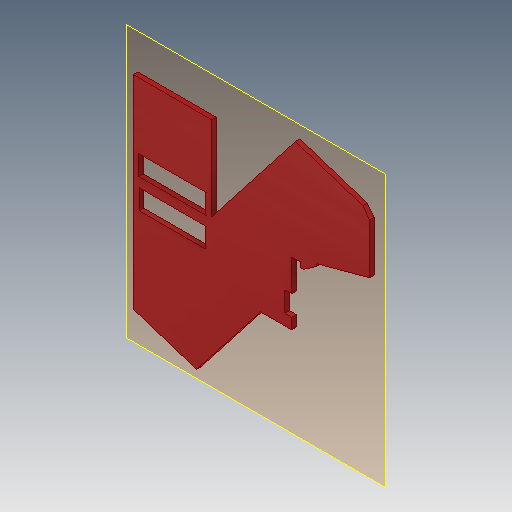
# Autodesk Inventor part: cellSTORM_v5_microscope_cover
Saved by Autodesk Inventor 2019.4 (Build 234330000, 330)
## iProperties
Created: 2020-04-27
Part Number: cellSTORM_v5_microscope_cover
Material: Generic
Document SubType Name: Modeling
Designer: diederichbenedict
Density: 1 g/cm^3
Appearance: Red
Author: diederichbenedict
Autodesk Inventor part; units mm, degrees
ref_plane "YZ Plane" through (0, 0, 0) normal (1, 0, 0) x (0, 1, 0)
ref_plane "XZ Plane" through (0, 0, 0) normal (0, 1, 0) x (-1, 0, 0)
ref_plane "XY Plane" through (0, 0, 0) normal (0, 0, 1) x (1, 0, 0)
ref_plane "Work Plane1" through (0, 0, 0) normal (0, 0, 1) x (1, 0, 0)
sketch "Sketch1" plane through (0, 0, 0) normal (0, 0, 1) x (1, 0, 0)
  line L0 (29.3421, 3.5361) -> (54.2162, 10.2011) projected
  line L1 (29.3421, 3.5361) -> (22.8734, 3.5361) projected
  line L2 (22.8734, 3.5361) -> (22.8734, -8.6704) projected
  line L3 (22.8734, -8.6704) -> (19.1468, -13.4402) projected
  line L4 (19.1468, -13.4402) -> (12.0348, -13.4402) projected
  line L5 (12.0348, -13.4402) -> (12.0348, -22.5432) projected
  line L6 (12.0348, -22.5432) -> (-14.689, -56.7481) projected
  line L7 (-14.689, -56.7481) -> (-41.2, -48.1342) projected
  line L8 (-41.2, -48.1342) -> (-41.2, -18.0876) projected
  line L9 (-41.2, -7.0876) -> (-38.2, -7.0876) projected
  line L10 (-38.2, -7.0876) -> (-38.2, -2.0876) projected
  line L11 (-38.2, -2.0876) -> (-41.4512, -2.0876) projected
  line L12 (-41.4512, -2.0876) -> (-41.4512, 5.4124) construction
  line L13 (-41.4512, 5.4124) -> (-41.2, 5.4124) construction
  line L14 (-41.2, 5.4124) -> (-41.2, 5.9124) construction
  line L15 (-41.2, 5.9124) -> (-38.2, 5.9124) projected
  line L16 (-38.2, 5.9124) -> (-38.2, 8.4124) projected
  line L17 (-38.2, 8.4124) -> (-41.2, 8.4124) projected
  line L18 (-41.2, 8.4124) -> (-41.2, 32.4124) projected
  line L19 (-41.2, 32.4124) -> (-12.4512, 32.4124) projected
  line L20 (-12.4512, 32.4124) -> (-12.4512, 8.4124) projected
  line L21 (-12.4512, 8.4124) -> (-15.4512, 8.4124) projected
  line L22 (-15.4512, 8.4124) -> (-15.4512, 5.9124) projected
  line L23 (-15.4512, 5.9124) -> (-12.4512, 5.9124) projected
  line L24 (-12.4512, 5.9124) -> (-12.4512, -2.0876) projected
  line L25 (-12.4512, -2.0876) -> (-15.4512, -2.0876) projected
  line L26 (-15.4512, -2.0876) -> (-15.4512, -7.0876) projected
  line L27 (-15.4512, -7.0876) -> (-12.4512, -7.0876) projected
  line L28 (-12.4512, -7.0876) -> (-12.4512, -15.0876) projected
  line L29 (-10.7358, -8.2808) -> (27.1735, 40.2407) projected
  line L30 (27.1735, 40.2407) -> (54.2162, 31.454) projected
  line L31 (54.2162, 31.454) -> (54.2162, 10.2011) projected
  line L32 (36.5437, 2.1484) -> (31.1264, -1.592) projected
  line L33 (36.5437, 2.1484) -> (37.0695, 3.5361) projected
  line L34 (60.3683, 9.779) -> (37.0695, 3.5361) projected
  line L35 (60.3683, 9.779) -> (60.3683, 9.784) projected
  line L36 (60.3683, 9.784) -> (60.3683, 25.084) projected
  line L37 (60.3683, 25.084) -> (60.3683, 31.9539) projected
  line L38 (60.3683, 31.9539) -> (57.3683, 35.9287) projected
  line L39 (57.3683, 35.9287) -> (27.5635, 45.6128) projected
  line L40 (27.5635, 45.6128) -> (-9.4512, -1.7639) projected
  line L41 (-9.4512, -1.7639) -> (-9.4512, 35.4124) projected
  line L42 (-9.4512, 35.4124) -> (-42.2, 35.4124) projected
  line L43 (-42.2, 35.4124) -> (-44.2, 35.4124) projected
  line L44 (-44.2, 35.4124) -> (-44.2, -54.5196) projected
  line L45 (-44.2, -54.5196) -> (-16.239, -63.6047) projected
  line L46 (-16.239, -63.6047) -> (12.0348, -27.416) projected
  line L47 (12.0348, -27.416) -> (25.8734, -27.416) projected
  line L48 (25.8734, -27.416) -> (25.8734, -22.5432) projected
  line L49 (25.8734, -22.5432) -> (22.8734, -22.5432) projected
  line L50 (22.8734, -22.5432) -> (22.8734, -13.5432) projected
  line L51 (22.8734, -13.5432) -> (25.8734, -13.5432) projected
  line L52 (25.8734, -13.5432) -> (25.8734, 0.5361) projected
  line L53 (25.8734, 0.5361) -> (29.5751, 0.5361) projected
  line L54 (29.5751, 0.5361) -> (29.5751, -1.592) projected
  line L55 (29.5751, -1.592) -> (31.1264, -1.592) projected
  line L56 (-12.4512, 5.9124) -> (-41.4512, 5.9124)
  line L57 (-41.4512, 5.9124) -> (-41.4512, -2.0876) construction
  line L58 (-41.4512, -2.0876) -> (-12.4512, -2.0876)
  line L59 (-12.4512, -2.0876) -> (-12.4512, 5.9124)
  line L60 (-12.4512, -7.0876) -> (-41.2, -7.0876)
  line L61 (-41.2, -7.0876) -> (-41.2, -15.0876)
  line L62 (-41.2, -15.0876) -> (-12.4512, -15.0876)
  line L63 (-12.4512, -15.0876) -> (-12.4512, -7.0876)
  line L64 (-41.4512, 5.9124) -> (-41.4512, -2.0876)
  line L65 (-41.2, -18.0876) -> (-38.2, -18.0876) projected
  line L66 (-38.2, -18.0876) -> (-38.2, -15.0876) projected
  line L67 (-38.2, -15.0876) -> (-41.2, -15.0876) projected
  line L68 (-41.2, -15.0876) -> (-41.2, -7.0876) projected
  line L69 (-12.4512, -15.0876) -> (-14.4512, -15.0876) projected
  line L70 (-14.4512, -15.0876) -> (-14.4512, -17.0876) projected
  line L71 (-14.4512, -17.0876) -> (-10.7358, -17.0876) projected
  line L72 (-10.7358, -17.0876) -> (-10.7358, -8.2808) projected
  point P0 (0, 0)
  dimension "d0" = 8
  constraints: 18 end point, 4 parallel, 2 horizontal, 2 perpendicular, 1 collinear, 1 point on line
  measures "d0" distance of L61.end L60.end
extrude "Extrusion1" add sketch "Sketch1" along normal blind 2 contours L1 L2 L3 L4 L5 L6 L7 L8 L65 L66 L62 L70 L71 L72 L29 L30 L31 L0 | L60 L10 L58 L26 | L56 L16 L17 L18 L19 L20 L21 L22 | L32 L55 L54 L53 L52 L51 L50 L49 L48 L47 L46 L45 L44 L43 L42 L41 L40 L39 L38 L37 L36 L35 L34 L33
sketch "Sketch2" plane through (0, 0, 0) normal (0, 0, -1) x (-1, 0, 0)
  line L0 (12.4512, -15.0876) -> (12.4512, -7.0876) projected
  line L1 (12.4512, -7.0876) -> (41.2, -7.0876) projected
  line L2 (41.2, -7.0876) -> (41.2, -15.0876) projected
  line L3 (41.2, -15.0876) -> (12.4512, -15.0876) projected
  line L4 (41.4512, 5.9124) -> (41.4512, -2.0876) projected
  line L5 (41.4512, -2.0876) -> (12.4512, -2.0876) projected
  line L6 (12.4512, -2.0876) -> (12.4512, 5.9124) projected
  line L7 (12.4512, 5.9124) -> (41.4512, 5.9124) projected
  line L8 (-36.5437, 2.1484) -> (-31.1264, -1.592) projected
  line L9 (-31.1264, -1.592) -> (-29.5751, -1.592) projected
  line L10 (-29.5751, -1.592) -> (-29.5751, 0.5361) projected
  line L11 (-29.5751, 0.5361) -> (-25.8734, 0.5361) projected
  line L12 (-25.8734, 0.5361) -> (-25.8734, -13.5432) projected
  line L13 (-25.8734, -13.5432) -> (-22.8734, -13.5432) projected
  line L14 (-22.8734, -13.5432) -> (-22.8734, -22.5432) projected
  line L15 (-22.8734, -22.5432) -> (-25.8734, -22.5432) projected
  line L16 (-25.8734, -22.5432) -> (-25.8734, -27.416) projected
  line L17 (-25.8734, -27.416) -> (-12.0348, -27.416) projected
  line L18 (-12.0348, -27.416) -> (16.239, -63.6047) projected
  line L19 (16.239, -63.6047) -> (44.2, -54.5196) projected
  line L20 (44.2, -54.5196) -> (44.2, 35.4124) projected
  line L21 (44.2, 35.4124) -> (9.4512, 35.4124) projected
  line L22 (9.4512, 35.4124) -> (9.4512, -1.7639) projected
  line L23 (9.4512, -1.7639) -> (-27.5635, 45.6128) projected
  line L24 (-27.5635, 45.6128) -> (-57.3683, 35.9287) projected
  line L25 (-57.3683, 35.9287) -> (-60.3683, 31.9539) projected
  line L26 (-60.3683, 31.9539) -> (-60.3683, 9.784) projected
  line L27 (-60.3683, 9.784) -> (-60.3683, 9.779) projected
  line L28 (-60.3683, 9.779) -> (-37.0695, 3.5361) projected
  line L29 (-37.0695, 3.5361) -> (-36.5437, 2.1484) projected
  line L30 (-29.3421, 3.5361) -> (-54.2162, 10.2011) projected
  line L31 (-54.2162, 10.2011) -> (-54.2162, 31.454) projected
  line L32 (-54.2162, 31.454) -> (-27.1735, 40.2407) projected
  line L33 (-27.1735, 40.2407) -> (10.7358, -8.2808) projected
  line L34 (12.4512, -15.0876) -> (12.4512, -7.0876) projected
  line L35 (12.4512, -7.0876) -> (15.4512, -7.0876) projected
  line L36 (15.4512, -7.0876) -> (15.4512, -2.0876) projected
  line L37 (15.4512, -2.0876) -> (12.4512, -2.0876) projected
  line L38 (12.4512, -2.0876) -> (12.4512, 5.9124) projected
  line L39 (12.4512, 5.9124) -> (15.4512, 5.9124) projected
  line L40 (15.4512, 5.9124) -> (15.4512, 8.4124) projected
  line L41 (15.4512, 8.4124) -> (12.4512, 8.4124) projected
  line L42 (12.4512, 8.4124) -> (12.4512, 32.4124) projected
  line L43 (12.4512, 32.4124) -> (41.2, 32.4124) projected
  line L44 (41.2, 32.4124) -> (41.2, 8.4124) projected
  line L45 (41.2, 8.4124) -> (38.2, 8.4124) projected
  line L46 (38.2, 8.4124) -> (38.2, 5.9124) projected
  line L47 (38.2, 5.9124) -> (41.2, 5.9124) projected
  line L48 (41.2, 5.9124) -> (41.2, 5.4124) projected
  line L49 (41.2, 5.4124) -> (41.4512, 5.4124) projected
  line L50 (41.4512, 5.4124) -> (41.4512, -2.0876) projected
  line L51 (41.4512, -2.0876) -> (38.2, -2.0876) projected
  line L52 (38.2, -2.0876) -> (38.2, -7.0876) projected
  line L53 (38.2, -7.0876) -> (41.2, -7.0876) projected
  line L54 (41.2, -18.0876) -> (41.2, -48.1342) projected
  line L55 (41.2, -48.1342) -> (14.689, -56.7481) projected
  line L56 (14.689, -56.7481) -> (-12.0348, -22.5432) projected
  line L57 (-12.0348, -22.5432) -> (-12.0348, -13.4402) projected
  line L58 (-12.0348, -13.4402) -> (-19.1468, -13.4402) projected
  line L59 (-19.1468, -13.4402) -> (-22.8734, -8.6704) projected
  line L60 (-22.8734, -8.6704) -> (-22.8734, 3.5361) projected
  line L61 (-22.8734, 3.5361) -> (-29.3421, 3.5361) projected
  circle A0 centre (37.2, 11.8299) radius 1.45 projected
  circle A1 centre (16.4512, 11.8299) radius 1.45 projected
  line L62 (12.6512, -7.0876) -> (12.6512, -11.0573)
  line L63 (12.6512, -11.0573) -> (-27.2448, 40.0073)
  line L64 (-27.2448, 40.0073) -> (-54.0162, 31.3087)
  line L65 (-54.0162, 31.3087) -> (-54.0162, 10.3546)
  line L66 (-54.0162, 10.3546) -> (-29.3158, 3.7361)
  line L67 (-29.3158, 3.7361) -> (-22.6734, 3.7361)
  line L68 (-22.6734, 3.7361) -> (-22.6734, -8.6016)
  line L69 (-22.6734, -8.6016) -> (-19.0493, -13.2402)
  line L70 (-19.0493, -13.2402) -> (-11.8348, -13.2402)
  line L71 (-11.8348, -13.2402) -> (-11.8348, -22.4744)
  line L72 (-11.8348, -22.4744) -> (14.7604, -56.5146)
  line L73 (14.7604, -56.5146) -> (41, -47.9889)
  line L74 (41, -47.9889) -> (41, -7.0876)
  line L75 (12.2936, -10.5996) -> (12.2936, -15.3176)
  line L76 (12.2936, -15.3176) -> (41, -15.3176)
  line L77 (12.6512, 32.3124) -> (41, 32.3124)
  line L78 (41, 32.3124) -> (41, 24.3283)
  line L79 (41, 24.3283) -> (12.6512, 24.3283)
  line L80 (12.6512, 24.3283) -> (12.6512, 32.3124)
  line L81 (41.2, -15.0876) -> (38.2, -15.0876) projected
  line L82 (38.2, -15.0876) -> (38.2, -18.0876) projected
  line L83 (38.2, -18.0876) -> (41.2, -18.0876) projected
  line L84 (10.7358, -8.2808) -> (10.7358, -17.0876) projected
  line L85 (10.7358, -17.0876) -> (14.4512, -17.0876) projected
  line L86 (14.4512, -17.0876) -> (14.4512, -15.0876) projected
  line L87 (14.4512, -15.0876) -> (12.4512, -15.0876) projected
  line L88 (41.2, -7.0876) -> (41.2, -15.0876) projected
  point P0 (0, 0)
  point P1 (12.4512, -10.4765)
  dimension "d3" = 0.2
  dimension "d4" = 7.9841
  dimension "d5" = 0.2
  dimension "d6" = 0.2
  dimension "d7" = 0.1
  constraints: 38 end point, 2 parallel, 2 perpendicular, 2 point on line, 1 horizontal, 1 vertical, 12 other
  measures "d3" distance between parallel lines of L31 L65
  measures "d4" distance of L79.end L77.start
  measures "d5" distance between parallel lines of L80 L42
  measures "d6" distance between parallel lines of L44 L78
  measures "d7" distance between parallel lines of L43 L77
extrude "Extrusion2" add sketch "Sketch2" along normal blind 2 contours L0 L63 L62 L1 L74 L3 | L0 L1 L62 L63 | L3 L82 L76 L86 | L76 L82 L83 L74 L73 L72 L71 L70 L69 L68 L67 L66 L65 L64 L63 L84 L85 L86 | L63 L64 L65 L66 L67 L68 L69 L70 L71 L72 L73 L74 L83 L54 L55 L56 L57 L58 L59 L60 L61 L30 L31 L32 L33 L84 | L74 L1 L2 L3 | L36 L5 L52 L1 | L77 L78 L79 L80
sketch "Sketch3" plane through (0, 0, -2) normal (0, 0, -1) x (-1, 0, 0)
  line L0 (12.4512, -7.0876) -> (12.4512, -15.0876) projected
  line L1 (10.7358, -8.2808) -> (-27.1735, 40.2407) projected
  line L2 (-27.1735, 40.2407) -> (-54.2162, 31.454) projected
  line L3 (-54.2162, 31.454) -> (-54.2162, 10.2011) projected
  line L4 (-54.2162, 10.2011) -> (-29.3421, 3.5361) projected
  line L5 (-29.3421, 3.5361) -> (-22.8734, 3.5361) projected
  line L6 (-22.8734, 3.5361) -> (-22.8734, -8.6704) projected
  line L7 (-22.8734, -8.6704) -> (-19.1468, -13.4402) projected
  line L8 (-19.1468, -13.4402) -> (-12.0348, -13.4402) projected
  line L9 (-12.0348, -13.4402) -> (-12.0348, -22.5432) projected
  line L10 (-12.0348, -22.5432) -> (14.689, -56.7481) projected
  line L11 (14.689, -56.7481) -> (41.2, -48.1342) projected
  line L12 (41.2, -15.0876) -> (41.2, -7.0876) projected
  line L13 (41.2, -7.0876) -> (38.2, -7.0876) projected
  line L14 (38.2, -7.0876) -> (38.2, -2.0876) projected
  line L15 (38.2, -2.0876) -> (15.4512, -2.0876) projected
  line L16 (15.4512, -2.0876) -> (15.4512, -7.0876) projected
  line L17 (15.4512, -7.0876) -> (12.4512, -7.0876) projected
  line L18 (38.2, -45.9545) -> (15.7598, -53.2458)
  line L19 (15.7598, -53.2458) -> (-9.0348, -21.5102)
  line L20 (-9.0348, -21.5102) -> (-9.0348, -10.4402)
  line L21 (-9.0348, -10.4402) -> (-17.6836, -10.4402)
  line L22 (-17.6836, -10.4402) -> (-19.8734, -7.6374)
  line L23 (-19.8734, -7.6374) -> (-19.8734, 6.5361)
  line L24 (-19.8734, 6.5361) -> (-28.9472, 6.5361)
  line L25 (-28.9472, 6.5361) -> (-51.2162, 12.5031)
  line L26 (-51.2162, 12.5031) -> (-51.2162, 29.2744)
  line L27 (-51.2162, 29.2744) -> (-28.2442, 36.7384)
  line L28 (-28.2442, 36.7384) -> (15.4512, -19.1891)
  line L29 (15.4512, -19.1891) -> (15.4512, -10.0876)
  line L30 (15.4512, -10.0876) -> (18.4512, -10.0876)
  line L31 (18.4512, -10.0876) -> (18.4512, -5.0876)
  line L32 (18.4512, -5.0876) -> (35.2, -5.0876)
  line L33 (35.2, -5.0876) -> (35.2, -10.0876)
  line L34 (35.2, -10.0876) -> (38.2, -10.0876)
  line L35 (38.2, -10.0876) -> (38.2, -45.9545)
  line L36 (12.4512, -15.0876) -> (14.4512, -15.0876) projected
  line L37 (14.4512, -15.0876) -> (14.4512, -17.0876) projected
  line L38 (14.4512, -17.0876) -> (10.7358, -17.0876) projected
  line L39 (10.7358, -17.0876) -> (10.7358, -8.2808) projected
  line L40 (41.2, -48.1342) -> (41.2, -18.0876) projected
  line L41 (41.2, -18.0876) -> (38.2, -18.0876) projected
  line L42 (38.2, -18.0876) -> (38.2, -15.0876) projected
  line L43 (38.2, -15.0876) -> (41.2, -15.0876) projected
  point P0 (0, 0)
  dimension "d10" = 3
  constraints: 36 end point, 17 other
  measures "d10" distance between parallel lines of L11 L18
extrude "Extrusion3" cut sketch "Sketch3" against normal up to surface (2 mm away) contours L38 L39 L28 | L28 L29 L30 L31 L32 L33 L34 L35 L18 L19 L20 L21 L22 L23 L24 L25 L26 L27 L39 L38
sketch "Sketch4" plane through (0, 0, 2) normal (0, 0, 1) x (1, 0, 0)
  line L0 (-12.4512, -7.0876) -> (-12.4512, -15.0876) projected
  line L1 (-12.4512, -15.0876) -> (-41.2, -15.0876) projected
  line L2 (-41.2, -15.0876) -> (-41.2, -7.0876) projected
  line L3 (-41.2, -7.0876) -> (-12.4512, -7.0876) projected
  line L4 (-41.4512, -2.0876) -> (-41.4512, 5.9124) projected
  line L5 (-41.4512, 5.9124) -> (-12.4512, 5.9124) projected
  line L6 (-12.4512, 5.9124) -> (-12.4512, -2.0876) projected
  line L7 (-12.4512, -2.0876) -> (-41.4512, -2.0876) projected
  line L8 (31.1264, -1.592) -> (36.5437, 2.1484) projected
  line L9 (36.5437, 2.1484) -> (37.0695, 3.5361) projected
  line L10 (37.0695, 3.5361) -> (60.3683, 9.779) projected
  line L11 (60.3683, 9.779) -> (60.3683, 9.784) projected
  line L12 (60.3683, 9.784) -> (60.3683, 31.9539) projected
  line L13 (60.3683, 31.9539) -> (57.3683, 35.9287) projected
  line L14 (57.3683, 35.9287) -> (27.5635, 45.6128) projected
  line L15 (27.5635, 45.6128) -> (-9.4512, -1.7639) projected
  line L16 (-9.4512, -1.7639) -> (-9.4512, 35.4124) projected
  line L17 (-9.4512, 35.4124) -> (-44.2, 35.4124) projected
  line L18 (-44.2, 35.4124) -> (-44.2, -54.5196) projected
  line L19 (-44.2, -54.5196) -> (-16.239, -63.6047) projected
  line L20 (-16.239, -63.6047) -> (12.0348, -27.416) projected
  line L21 (12.0348, -27.416) -> (25.8734, -27.416) projected
  line L22 (25.8734, -27.416) -> (25.8734, -22.5432) projected
  line L23 (25.8734, -22.5432) -> (22.8734, -22.5432) projected
  line L24 (22.8734, -22.5432) -> (22.8734, -13.5432) projected
  line L25 (22.8734, -13.5432) -> (25.8734, -13.5432) projected
  line L26 (25.8734, -13.5432) -> (25.8734, 0.5361) projected
  line L27 (25.8734, 0.5361) -> (29.5751, 0.5361) projected
  line L28 (29.5751, 0.5361) -> (29.5751, -1.592) projected
  line L29 (29.5751, -1.592) -> (31.1264, -1.592) projected
  line L30 (-41.6, -6.6876) -> (-41.6, -15.4876)
  line L31 (-41.6, -15.4876) -> (-12.0512, -15.4876)
  line L32 (-12.0512, -15.4876) -> (-12.0512, -6.6876)
  line L33 (-12.0512, -6.6876) -> (-41.6, -6.6876)
  line L34 (-41.8512, 6.3124) -> (-41.8512, -2.4876)
  line L35 (-41.8512, -2.4876) -> (-12.0512, -2.4876)
  line L36 (-12.0512, -2.4876) -> (-12.0512, 6.3124)
  line L37 (-12.0512, 6.3124) -> (-41.8512, 6.3124)
  point P0 (0, 0)
  dimension "d13" = 0.4
  dimension "d14" = 0.4
  constraints: 16 end point, 6 other
  measures "d13" distance between parallel lines of L2 L30
  measures "d14" distance between parallel lines of L4 L34
extrude "Extrusion4" cut sketch "Sketch4" against normal through all contours L0 L1 L2 L3 | L4 L5 L6 L7 | L33 L32 L31 L30 | L37 L36 L35 L34
sketch "Sketch5" plane through (28.9472, 6.5361, 0) normal (0, 0, -1) x (-1, 0, 0)
  line L0 (40.9984, -22.0237) -> (40.9984, -13.2237) projected
  line L1 (44.3984, -25.7253) -> (42.7564, -23.6237) projected
  line L2 (0.703, 30.2023) -> (-22.269, 22.7383) projected
  line L3 (-22.269, 22.7383) -> (-22.269, 5.967) projected
  line L4 (-22.269, 5.967) -> (0, 0) projected
  line L5 (0, 0) -> (9.0738, 0) projected
  line L6 (9.0738, 0) -> (9.0738, -14.1736) projected
  line L7 (9.0738, -14.1736) -> (11.2636, -16.9764) projected
  line L8 (11.2636, -16.9764) -> (19.9124, -16.9764) projected
  line L9 (19.9124, -16.9764) -> (19.9124, -28.0464) projected
  line L10 (19.9124, -28.0464) -> (44.707, -59.7819) projected
  line L11 (44.707, -59.7819) -> (67.1472, -52.4907) projected
  line L12 (67.1472, -52.4907) -> (67.1472, -24.6237) projected
  line L13 (43.3984, -22.0237) -> (40.9984, -22.0237) projected
  line L14 (44.3984, -22.0237) -> (44.3984, -25.7253) projected
  line L15 (39.6829, -19.6898) -> (0.703, 30.2023) projected
  line L16 (70.5472, -22.0237) -> (44.3984, -22.0237) projected
  line L17 (82.7759, -30.6849) -> (35.5398, -30.6849)
  line L18 (35.5398, -30.6849) -> (35.5398, 1.4585)
  line L19 (35.5398, 1.4585) -> (82.7759, 1.4585)
  line L20 (82.7759, 1.4585) -> (82.7759, -30.6849)
  line L21 (40.9984, -13.2237) -> (44.3984, -13.2237) projected
  line L22 (44.3984, -13.2237) -> (44.3984, -9.0237) projected
  line L23 (44.3984, -9.0237) -> (40.9984, -9.0237) projected
  line L24 (40.9984, -9.0237) -> (40.9984, -0.2237) projected
  line L25 (40.9984, -0.2237) -> (70.7984, -0.2237) projected
  line L26 (70.7984, -0.2237) -> (70.7984, -9.0237) projected
  line L27 (70.7984, -9.0237) -> (67.1472, -9.0237) projected
  line L28 (67.1472, -9.0237) -> (67.1472, -13.2237) projected
  line L29 (67.1472, -13.2237) -> (70.5472, -13.2237) projected
  line L30 (70.5472, -13.2237) -> (70.5472, -22.0237) projected
  line L31 (42.7564, -23.6237) -> (43.3984, -23.6237) projected
  line L32 (43.3984, -23.6237) -> (43.3984, -22.0237) projected
  line L33 (67.1472, -24.6237) -> (70.1472, -24.6237) projected
  line L34 (70.1472, -24.6237) -> (70.1472, -54.6703) projected
  line L35 (70.1472, -54.6703) -> (43.6362, -63.2842) projected
  line L36 (43.6362, -63.2842) -> (16.9124, -29.0794) projected
  line L37 (16.9124, -29.0794) -> (16.9124, -19.9764) projected
  line L38 (16.9124, -19.9764) -> (9.8004, -19.9764) projected
  line L39 (9.8004, -19.9764) -> (6.0738, -15.2066) projected
  line L40 (6.0738, -15.2066) -> (6.0738, -3) projected
  line L41 (6.0738, -3) -> (-0.395, -3) projected
  line L42 (-0.395, -3) -> (-25.269, 3.665) projected
  line L43 (-25.269, 3.665) -> (-25.269, 24.9179) projected
  line L44 (-25.269, 24.9179) -> (1.7737, 33.7046) projected
  line L45 (1.7737, 33.7046) -> (39.6829, -14.817) projected
  line L46 (39.6829, -14.817) -> (39.6829, -19.6898) projected
  point P0 (28.9472, -6.5361)
  constraints: 8 end point, 2 parallel, 1 horizontal, 1 perpendicular
extrude "Extrusion5" cut sketch "Sketch5" along normal blind 10 contours L0 L21 L22 L23 L24 L25 L26 L27 L28 L29 L30 L16 L14 L1 L31 L32 L13 | L18 L45 L46 L15 | L15 L46 L45 L18 L19 L20 L17 L34 L33 L12 | L12 L33 L34 L17
body "Solid1"
